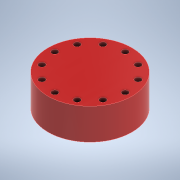
# Autodesk Inventor part: topAttachementForPvcPipe
Saved by Autodesk Inventor 2022.2 (Build 262287000, 287)
## iProperties
Created: 2021-10-20
Part Number: topAttachementForPvcPipe
Material: PC/ABS Plastic
Document SubType Name: Modeling
Designer: robst
Density: 0.357273 g/cm^3
Appearance: Red
Author: robst
Autodesk Inventor part; units mm, degrees
ref_plane "YZ Plane" through (0, 0, 0) normal (1, 0, 0) x (0, 1, 0)
ref_plane "XZ Plane" through (0, 0, 0) normal (0, 1, 0) x (-1, 0, 0)
ref_plane "XY Plane" through (0, 0, 0) normal (0, 0, 1) x (1, 0, 0)
sketch "Sketch51" plane through (0, 0, 0) normal (0, 1, 0) x (-1, 0, 0)
  circle A0 centre (0, 0) radius 44.45
  dimension "d242" = 88.9
  constraints: 1 centre point, 1 coincident
  measures "d242" diameter of A0
extrude "Extrusion26" add sketch "Sketch51" against normal blind 8
sketch "Sketch57" plane through (0, -8, 0) normal (0, -1, 0) x (1, 0, 0)
  circle A0 centre (0, 0) radius 26.2509
  circle A1 centre (0, 0) radius 30.1625
  circle A2 centre (0, 0) radius 44.45 projected
  circle A3 centre (0, 0) radius 44.45
  dimension "d290" = 52.5018
  dimension "d291" = 60.325
  constraints: 3 centre point, 3 coincident, 1 concentric
  measures "d290" diameter of A0
  measures "d291" diameter of A1
extrude "Extrusion28" add sketch "Sketch57" along normal blind 25
sketch "Sketch58" plane through (0, 0, 0) normal (0, 1, 0) x (1, 0, 0)
  point P0 (0, 0)
  point P1 (0, 37.3063)
  point P2 (-18.6531, 32.3082)
  point P3 (-32.3082, 18.6531)
  point P4 (-37.3063, 0)
  point P5 (-32.3082, -18.6531)
  point P6 (-18.6531, -32.3082)
  point P7 (0, -37.3063)
  point P8 (18.6531, -32.3082)
  point P9 (32.3082, -18.6531)
  point P10 (37.3063, 0)
  point P11 (32.3082, 18.6531)
  point P12 (18.6531, 32.3082)
  dimension "d294" = 37.3062
  dimension "d297" = 360
  constraints: 13 other
  measures "d294" distance of point (0, 37.306) point (0, 0)
hole "Hole9" at (0, 0, -37.3063) at (-18.6531, 0, -32.3082) at (-32.3082, 0, -18.6531) at (-37.3063, 0, 0) at (-32.3082, 0, 18.6531) at (-18.6531, 0, 32.3082) at (0, 0, 37.3063) at (18.6531, 0, 32.3082) at (32.3082, 0, 18.6531) at (37.3063, 0, 0) at (32.3082, 0, -18.6531) at (18.6531, 0, -32.3082) direction (0, -1, 0) diameter 5.105 end through all counterbore diameter 6.3754 counterbore depth 9.525 clearance for "Hex Machine Screw" size "#10" standard "Ansi Unified Screw Threads"
equation "\"d242\" = outsideDiameterOfBottom"
equation "\"d243\" = wallThickness"
equation "\"d290\" = pvc2InchPipeInsideDiameter"
equation "\"d291\" = pvc2InchPipeOutsideDiameter"
equation "\"d292\" = pvcPipeInsertDepth"
equation "\"wallThickness\" = 8"
equation "\"twoByFourWidth\" = 40.64"
equation "\"twoByFourDepth\" = 84.1375"
equation "\"azimuth\" = 55deg"
equation "\"elevationOfTwoByFour\" = 20deg"
equation "\"depthOfExtrusionForMatingToLowerHalf\" = 12.5"
equation "\"depthForWasherForMatingToCase\" = 14"
equation "\"pvc2InchPipeInsideDiameter\" = 52.5018"
equation "\"pvc2InchPipeOutsideDiameter\" = 60.325"
equation "\"pvcPipeInsertDepth\" = 25"
equation "\"outsideDiameterOfBottom\" = 88.9"
body "Solid4"
